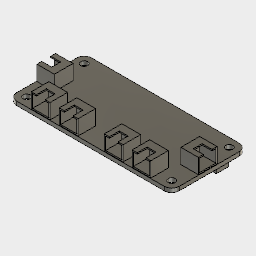
3422 Adafruit Arcade Bonnet (Autodesk Fusion 360 design; units mm, degrees)
Autodesk Fusion 360 part; units mm, degrees
sketch "Adafruit Arcade Bonnet" plane through (0, 0, 0) normal (0, 0, 1) x (1, 0, 0)
  circle A0 centre (3.5, 26.5) radius 1.4
  arc A1 (65, 27) -> (62, 30) centre (62, 27) ccw
  line L0 (65, 3) -> (65, 27)
  line L1 (62, 30) -> (3, 30)
  line L2 (0, 27) -> (0, 3)
  arc A2 (0, 3) -> (3, 0) centre (3, 3) ccw
  arc A3 (3, 30) -> (0, 27) centre (3, 27) ccw
  line L3 (3, 0) -> (62, 0)
  circle A4 centre (61.5, 26.5) radius 1.4
  circle A5 centre (3.5, 3.5) radius 1.4
  arc A6 (62, 0) -> (65, 3) centre (62, 3) ccw
  circle A7 centre (61.5, 3.5) radius 1.4
extrude "Extrude1" add sketch "Adafruit Arcade Bonnet" along normal blind 1.6 makes body 1
sketch "jst boxes" plane through (0, 0, 1.6) normal (0, 0, 1) x (-1, 0, 0)
  circle A0 centre (-3.5, -3.5) radius 1.4
  circle A1 centre (-61.5, -26.5) radius 1.4
  circle A2 centre (-61.5, -3.5) radius 1.4
  circle A3 centre (-3.5, -26.5) radius 1.4
  arc A4 (-62, 0) -> (-65, -3) centre (-62, -3) ccw
  line L0 (-65, -3) -> (-65, -27)
  arc A5 (-65, -27) -> (-62, -30) centre (-62, -27) ccw
  line L1 (-62, -30) -> (-3, -30)
  arc A6 (-3, -30) -> (0, -27) centre (-3, -27) ccw
  line L2 (0, -27) -> (0, -3)
  arc A7 (0, -3) -> (-3, 0) centre (-3, -3) ccw
  line L3 (-3, 0) -> (-62, 0)
  line L4 (-7.2, -10.85) -> (-0.2, -10.85)
  line L5 (-0.2, -10.85) -> (-0.2, -18.35)
  line L6 (-0.2, -18.35) -> (-7.2, -18.35)
  line L7 (-7.2, -18.35) -> (-7.2, -10.85)
  line L8 (-7.2, -10.85) -> (-0.2, -18.35) construction
  line L9 (-0.2, -10.85) -> (-7.2, -18.35) construction
  line L10 (-16.15, -0.2) -> (-8.65, -0.2)
  line L11 (-8.65, -0.2) -> (-8.65, -7.2)
  line L12 (-8.65, -7.2) -> (-16.15, -7.2)
  line L13 (-16.15, -7.2) -> (-16.15, -0.2)
  line L14 (-16.15, -0.2) -> (-8.65, -7.2) construction
  line L15 (-8.65, -0.2) -> (-16.15, -7.2) construction
  line L16 (-27.35, -0.2) -> (-19.85, -0.2)
  line L17 (-19.85, -0.2) -> (-19.85, -7.2)
  line L18 (-19.85, -7.2) -> (-27.35, -7.2)
  line L19 (-27.35, -7.2) -> (-27.35, -0.2)
  line L20 (-27.35, -0.2) -> (-19.85, -7.2) construction
  line L21 (-19.85, -0.2) -> (-27.35, -7.2) construction
  line L22 (-56.45, -0.2) -> (-48.95, -0.2)
  line L23 (-48.95, -0.2) -> (-48.95, -7.2)
  line L24 (-48.95, -7.2) -> (-56.45, -7.2)
  line L25 (-56.45, -7.2) -> (-56.45, -0.2)
  line L26 (-56.45, -0.2) -> (-48.95, -7.2) construction
  line L27 (-48.95, -0.2) -> (-56.45, -7.2) construction
  line L28 (-45.35, -0.2) -> (-37.85, -0.2)
  line L29 (-37.85, -0.2) -> (-37.85, -7.2)
  line L30 (-37.85, -7.2) -> (-45.35, -7.2)
  line L31 (-45.35, -7.2) -> (-45.35, -0.2)
  line L32 (-45.35, -0.2) -> (-37.85, -7.2) construction
  line L33 (-37.85, -0.2) -> (-45.35, -7.2) construction
  line L34 (-64.8, -10.85) -> (-57.8, -10.85)
  line L35 (-57.8, -10.85) -> (-57.8, -18.35)
  line L36 (-57.8, -18.35) -> (-64.8, -18.35)
  line L37 (-64.8, -18.35) -> (-64.8, -10.85)
  line L38 (-64.8, -10.85) -> (-57.8, -18.35) construction
  line L39 (-57.8, -10.85) -> (-64.8, -18.35) construction
  point P0 (-3.7, -14.6)
  point P1 (-12.4, -3.7)
  point P2 (-23.6, -3.7)
  point P3 (-52.7, -3.7)
  point P4 (-41.6, -3.7)
  point P5 (-61.3, -14.6)
  dimension "d3" = 7.5
  dimension "d4" = 7
  dimension "d5" = 14.6
  dimension "d6" = 0.2
  dimension "d7" = 7.5
  dimension "d8" = 7
  dimension "d9" = 12.4
  dimension "d10" = 0.2
  dimension "d11" = 7.5
  dimension "d12" = 7
  dimension "d13" = 23.6
  dimension "d14" = 0.2
  dimension "d15" = 7.5
  dimension "d16" = 7
  dimension "d17" = 52.7
  dimension "d18" = 0.2
  dimension "d19" = 7.5
  dimension "d20" = 7
  dimension "d21" = 41.6
  dimension "d22" = 0.2
  dimension "d23" = 7.5
  dimension "d24" = 7
  dimension "d25" = 14.6
  dimension "d26" = 0.2
  measures "d3" distance of L4.end L5.end
  measures "d4" distance of L5.end L6.end
  measures "d5" distance of L3 P0
  measures "d6" distance of L2 L5
  measures "d7" distance of L11.end L12.end
  measures "d8" distance of L10.end L11.end
  measures "d9" distance of L2 P1
  measures "d10" distance of L3 L10
  measures "d11" distance of L17.end L18.end
  measures "d12" distance of L16.end L17.end
  measures "d13" distance of L2 P2
  measures "d14" distance of L3 L16
  measures "d15" distance of L23.end L24.end
  measures "d16" distance of L22.end L23.end
  measures "d17" distance of L2 P3
  measures "d18" distance of L3 L22
  measures "d19" distance of L29.end L30.end
  measures "d20" distance of L28.end L29.end
  measures "d21" distance of L2 P4
  measures "d22" distance of L3 L28
  measures "d23" distance of L34.end L35.end
  measures "d24" distance of L35.end L36.end
  measures "d25" distance of L3 P5
  measures "d26" distance of L0 L37
extrude "Extrude2" add sketch "jst boxes" along normal blind 6 separate body contours L4 L5 L6 L7 | L10 L11 L12 L13 | L16 L17 L18 L19 | L22 L23 L24 L25 | L28 L29 L30 L31 | L34 L35 L36 L37 makes body 2 at (40.35, 2.5333, 1.6) makes body 3 at (4.8667, 13.35, 1.6) makes body 4 at (53.95, 2.5333, 1.6) makes body 5 at (24.85, 2.5333, 1.6) makes body 6 at (13.65, 4.8667, 1.6) makes body 7 at (60.1333, 15.85, 1.6)
sketch "jst cuts" plane through (0, 0, 7.6) normal (0, 0, 1) x (-1, 0, 0)
  line L0 (-7.2, -18.35) -> (-0.2, -18.35)
  line L1 (-0.2, -18.35) -> (-0.2, -10.85)
  line L2 (-0.2, -10.85) -> (-7.2, -10.85)
  line L3 (-7.2, -10.85) -> (-7.2, -18.35)
  line L4 (-16.15, -7.2) -> (-8.65, -7.2)
  line L5 (-8.65, -7.2) -> (-8.65, -0.2)
  line L6 (-8.65, -0.2) -> (-16.15, -0.2)
  line L7 (-16.15, -0.2) -> (-16.15, -7.2)
  line L8 (-27.35, -7.2) -> (-19.85, -7.2)
  line L9 (-19.85, -7.2) -> (-19.85, -0.2)
  line L10 (-19.85, -0.2) -> (-27.35, -0.2)
  line L11 (-27.35, -0.2) -> (-27.35, -7.2)
  line L12 (-45.35, -7.2) -> (-37.85, -7.2)
  line L13 (-37.85, -7.2) -> (-37.85, -0.2)
  line L14 (-37.85, -0.2) -> (-45.35, -0.2)
  line L15 (-45.35, -0.2) -> (-45.35, -7.2)
  line L16 (-56.45, -7.2) -> (-48.95, -7.2)
  line L17 (-48.95, -7.2) -> (-48.95, -0.2)
  line L18 (-48.95, -0.2) -> (-56.45, -0.2)
  line L19 (-56.45, -0.2) -> (-56.45, -7.2)
  line L20 (-64.8, -18.35) -> (-57.8, -18.35)
  line L21 (-57.8, -18.35) -> (-57.8, -10.85)
  line L22 (-57.8, -10.85) -> (-64.8, -10.85)
  line L23 (-64.8, -10.85) -> (-64.8, -18.35)
  line L24 (-4.2, -12.85) -> (3.8, -12.85)
  line L25 (3.8, -12.85) -> (3.8, -16.35)
  line L26 (3.8, -16.35) -> (-4.2, -16.35)
  line L27 (-4.2, -16.35) -> (-4.2, -12.85)
  line L28 (-4.2, -12.85) -> (3.8, -16.35) construction
  line L29 (3.8, -12.85) -> (-4.2, -16.35) construction
  line L30 (-14.15, 3.8) -> (-10.65, 3.8)
  line L31 (-10.65, 3.8) -> (-10.65, -4.2)
  line L32 (-10.65, -4.2) -> (-14.15, -4.2)
  line L33 (-14.15, -4.2) -> (-14.15, 3.8)
  line L34 (-14.15, 3.8) -> (-10.65, -4.2) construction
  line L35 (-10.65, 3.8) -> (-14.15, -4.2) construction
  line L36 (-25.35, 3.8) -> (-21.85, 3.8)
  line L37 (-21.85, 3.8) -> (-21.85, -4.2)
  line L38 (-21.85, -4.2) -> (-25.35, -4.2)
  line L39 (-25.35, -4.2) -> (-25.35, 3.8)
  line L40 (-25.35, 3.8) -> (-21.85, -4.2) construction
  line L41 (-21.85, 3.8) -> (-25.35, -4.2) construction
  line L42 (-43.35, 3.8) -> (-39.85, 3.8)
  line L43 (-39.85, 3.8) -> (-39.85, -4.2)
  line L44 (-39.85, -4.2) -> (-43.35, -4.2)
  line L45 (-43.35, -4.2) -> (-43.35, 3.8)
  line L46 (-43.35, 3.8) -> (-39.85, -4.2) construction
  line L47 (-39.85, 3.8) -> (-43.35, -4.2) construction
  line L48 (-54.45, 3.8) -> (-50.95, 3.8)
  line L49 (-50.95, 3.8) -> (-50.95, -4.2)
  line L50 (-50.95, -4.2) -> (-54.45, -4.2)
  line L51 (-54.45, -4.2) -> (-54.45, 3.8)
  line L52 (-54.45, 3.8) -> (-50.95, -4.2) construction
  line L53 (-50.95, 3.8) -> (-54.45, -4.2) construction
  line L54 (-68.8, -12.85) -> (-60.8, -12.85)
  line L55 (-60.8, -12.85) -> (-60.8, -16.35)
  line L56 (-60.8, -16.35) -> (-68.8, -16.35)
  line L57 (-68.8, -16.35) -> (-68.8, -12.85)
  line L58 (-68.8, -12.85) -> (-60.8, -16.35) construction
  line L59 (-60.8, -12.85) -> (-68.8, -16.35) construction
  point P0 (-0.2, -14.6)
  point P1 (-12.4, -0.2)
  point P2 (-23.6, -0.2)
  point P3 (-41.6, -0.2)
  point P4 (-52.7, -0.2)
  point P5 (-64.8, -14.6)
  dimension "d31" = 8
  dimension "d32" = 3.5
  dimension "d33" = 3.5
  dimension "d34" = 8
  dimension "d35" = 8
  dimension "d36" = 3.5
  dimension "d37" = 8
  dimension "d38" = 3.5
  dimension "d39" = 8
  dimension "d40" = 3.5
  dimension "d41" = 8
  dimension "d42" = 3.5
  measures "d31" distance of L24.start L24.end
  measures "d32" distance of L24.end L25.end
  measures "d33" distance of L30.start L30.end
  measures "d34" distance of L30.end L31.end
  measures "d35" distance of L36.end L37.end
  measures "d36" distance of L37.end L38.end
  measures "d37" distance of L42.end L43.end
  measures "d38" distance of L43.end L44.end
  measures "d39" distance of L48.end L49.end
  measures "d40" distance of L49.end L50.end
  measures "d41" distance of L55.end L56.end
  measures "d42" distance of L54.end L55.end
shell "Shell1" thickness 0.5 removed faces 6 at (42.85, 0.2, 3.6) at (0.2, 13.35, 3.6) at (53.95, 0.2, 3.6) at (24.85, 0.2, 3.6) at (13.65, 0.2, 3.6) at (64.8, 15.85, 3.6) on bodies 2 3 4 5 6 7
extrude "Extrude3" cut sketch "jst cuts" against normal blind 0.5 contours L1 L24 L26 L27 | L6 L31 L32 L33 | L10 L37 L38 L39 | L14 L43 L44 L45 | L18 L49 L50 L51 | L23 L54 L55 L56 bodies 2 3 4 5 6 7
sketch "Sketch4" plane through (0, 0, 0) normal (0, 0, -1) x (1, 0, 0)
  circle A0 centre (3.5, -3.5) radius 1.4
  circle A1 centre (61.5, -26.5) radius 1.4
  circle A2 centre (61.5, -3.5) radius 1.4
  circle A3 centre (3.5, -26.5) radius 1.4
  arc A4 (65, -3) -> (62, 0) centre (62, -3) ccw
  line L0 (62, 0) -> (3, 0)
  arc A5 (3, 0) -> (0, -3) centre (3, -3) ccw
  line L1 (0, -3) -> (0, -27)
  arc A6 (0, -27) -> (3, -30) centre (3, -27) ccw
  line L2 (3, -30) -> (62, -30)
  arc A7 (62, -30) -> (65, -27) centre (62, -27) ccw
  line L3 (65, -27) -> (65, -3)
  line L4 (32.5, 0) -> (32.5, -30) construction
  line L5 (58, -29.8) -> (7, -29.8)
  line L6 (7, -29.8) -> (7, -24.8)
  line L7 (7, -24.8) -> (58, -24.8)
  line L8 (58, -24.8) -> (58, -29.8)
  line L9 (58, -29.8) -> (7, -24.8) construction
  line L10 (7, -29.8) -> (58, -24.8) construction
  point P0 (32.5, -27.3)
  dimension "d46" = 51
  dimension "d47" = 5
  dimension "d51" = 0.2
  measures "d46" distance of L6.end L7.end
  measures "d47" distance of L5.end L6.end
  measures "d51" distance of L2 L5
extrude "Extrude4" add sketch "Sketch4" along normal blind 8.5 contours L5 L6 L7 L8 bodies 1
equation "d3 = jstWidth"
equation "d4 = jstLeng"
equation "d7 = jstWidth"
equation "d8 = jstLeng"
equation "d11 = jstWidth"
equation "d12 = jstLeng"
equation "d15 = jstWidth"
equation "d16 = jstLeng"
equation "d19 = jstWidth"
equation "d20 = jstLeng"
equation "d23 = jstWidth"
equation "d24 = jstLeng"
equation "jstWidth = 7.5 mm"
equation "jstLeng = 7 mm"
